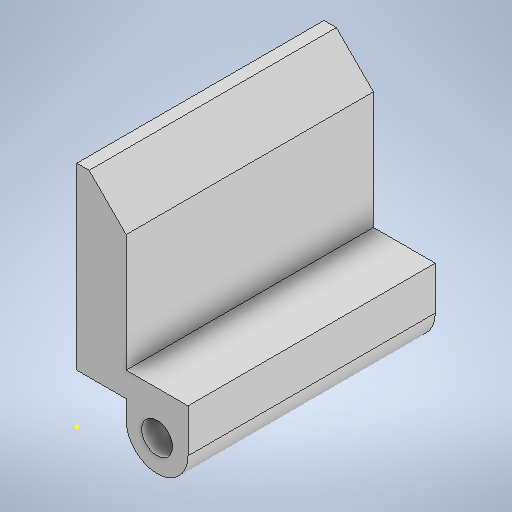
# Autodesk Inventor part: Hinge
Saved by Autodesk Inventor 2025 (Build 290162010, 162A)
## iProperties
Created: 2024-06-18
Part Number: Hinge
Material: Generic
Document SubType Name: Modeling
Designer: Alan Thomas
Mass: 12.1454 g
Surface Area: 53.2332 cm^2
Volume: 12.1454 cm^3
Density: 1 g/cm^3
Appearance: Default
Author: Alan Thomas
Autodesk Inventor part; units mm, degrees
ref_plane "YZ Plane" through (0, 0, 0) normal (1, 0, 0) x (0, 1, 0)
ref_plane "XZ Plane" through (0, 0, 0) normal (0, 1, 0) x (-1, 0, 0)
ref_plane "XY Plane" through (0, 0, 0) normal (0, 0, 1) x (1, 0, 0)
sketch "Sketch1" plane through (0, 0, 0) normal (0, 0, 1) x (1, 0, 0)
  line L0 (0, 0) -> (18, 0)
  line L1 (18, 0) -> (18, 32)
  line L2 (18, 32) -> (0, 32)
  line L3 (0, 32) -> (0, 0)
  dimension "d0" = 18
  dimension "d1" = 32
  constraints: 8 end point, 2 parallel, 1 horizontal, 1 perpendicular
  measures "d0" distance of L2.end L1.end
  measures "d1" distance of L1.end L0.end
extrude "Extrusion1" add sketch "Sketch1" along normal blind 40
sketch "Sketch2" plane through (0, 0, 40) normal (0, 0, 1) x (1, 0, 0)
  point P0 (0, 0)
sketch "Sketch3" plane through (0, 32, 0) normal (0, 1, 0) x (1, 0, 0)
  line L0 (18, -40) -> (8, -40)
  line L1 (8, -40) -> (8, 0)
  line L2 (8, 0) -> (18, 0)
  line L3 (18, 0) -> (18, -40)
  point P0 (0, 0)
  dimension "d4" = 10
  dimension "d5" = 40
  constraints: 8 end point, 2 parallel, 1 horizontal, 1 perpendicular
  measures "d4" distance of L1.end L2.end
  measures "d5" distance of L0.end L1.end
extrude "Extrusion2" cut sketch "Sketch3" against normal blind 20
sketch "Sketch4" plane through (0, 0, 40) normal (0, 0, 1) x (1, 0, 0)
  line L0 (0, 32) -> (0, 0) projected
  line L1 (0, 0) -> (8, 0)
  line L2 (8, 0) -> (8, 8)
  line L3 (8, 8) -> (0, 8)
  line L4 (0, 8) -> (0, 0)
  dimension "d8" = 8
  dimension "d9" = 8
  constraints: 8 end point, 2 parallel, 1 horizontal, 1 perpendicular
  measures "d8" distance of L3.end L2.end
  measures "d9" distance of L2.end L1.end
extrude "Extrusion3" cut sketch "Sketch4" against normal blind 40
fillet "Fillet1" radius 5 2 edges at (18, 0, 20) (8, 0, 20)
sketch "Sketch5" plane through (0, 0, 40) normal (0, 0, 1) x (1, 0, 0)
  arc A0 (8, 5) -> (18, 5) centre (13, 5) ccw projected
  circle A1 centre (13, 5) radius 2.5
  point P0 (0, 0)
  dimension "d13" = 5
  constraints: 1 centre point, 1 coincident
  measures "d13" diameter of A1
extrude "Extrusion4" cut sketch "Sketch5" against normal blind 40
sketch "Sketch6" plane through (0, 32, 40) normal (0, 1, 0) x (1, 0, 0)
  line L0 (0, 0) -> (8, 0) projected
  line L1 (8, 0) -> (8, 40) projected
  line L2 (0, 0) -> (8, 0)
  line L3 (8, 0) -> (8, 40)
  line L4 (8, 40) -> (0, 40)
  line L5 (0, 40) -> (0, 0)
  constraints: 8 end point, 2 parallel, 1 horizontal, 1 perpendicular
extrude "Extrusion5" add sketch "Sketch6" along normal blind 5
sketch "Sketch7" plane through (0, 0, 40) normal (0, 0, 1) x (1, 0, 0)
  line L0 (8, 37) -> (0, 37) projected
  line L1 (2, 37) -> (8, 31)
  line L2 (8, 37) -> (8, 12) projected
  point P0 (0, 0)
  dimension "d18" = 6
  constraints: 2 end point, 2 point on line
  measures "d18" horizontal distance of L1.start L1.end
extrude "Extrusion6" cut sketch "Sketch7" against normal blind 40
body "Solid1"
